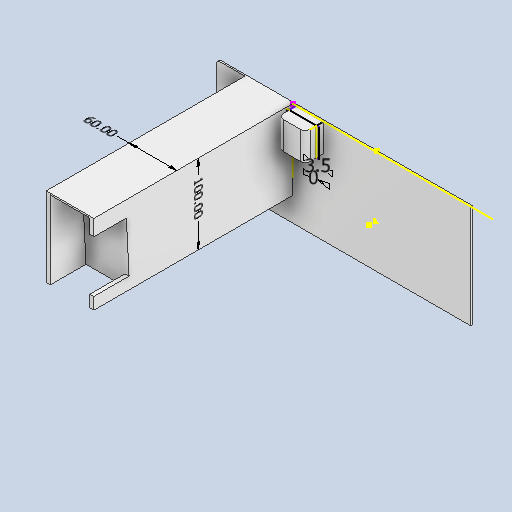
# Autodesk Inventor part: lifting base
Saved by Autodesk Inventor 2025.4 (Build 294407000, 407)
## iProperties
Created: 2026-03-06
Part Number: lifting base
Material: PPS Plastic
Document SubType Name: Modeling
Designer: eslam
Density: 1.637 g/cm^3
Appearance: Smooth - White
Mass: 2489.39 g
Surface Area: 2288.15 cm^2
Volume: 1520.71 cm^3
Author: eslam
Autodesk Inventor part; units mm, degrees
ref_plane "YZ Plane" through (0, 0, 0) normal (1, 0, 0) x (0, 1, 0)
ref_plane "XZ Plane" through (0, 0, 0) normal (0, 1, 0) x (-1, 0, 0)
sketch "Sketch1" plane through (0, 0, 0) normal (0, 0, 1) x (1, 0, 0)
  line L0 (200, 75) -> (-200, 75)
  line L1 (-200, 75) -> (-200, -75)
  line L2 (-200, -75) -> (200, -75)
  line L3 (200, -75) -> (200, 75)
  line L4 (200, 75) -> (-200, -75) construction
  line L5 (-200, 75) -> (200, -75) construction
  point P0 (0, 0)
  dimension "d0" = 400
  dimension "d1" = 150
  constraints: 12 end point, 2 midpoint, 2 parallel, 1 horizontal, 1 perpendicular
  measures "d0" distance of L2.end L1.end
  measures "d1" distance of L1.end L0.end
extrude "Extrusion1" add sketch "Sketch1" along normal blind 2
sketch "Sketch2" plane through (0, 0, 2) normal (0, 0, 1) x (1, 0, 0)
  line L0 (-200, 0) -> (-155, 56.4222) construction
  line L1 (-155, -56.4222) -> (-200, 0) construction
  line L2 (-104.6282, 75) -> (-164.6282, 75)
  line L3 (-164.6282, 75) -> (-164.6282, -25)
  line L4 (-164.6282, -25) -> (-104.6282, -25)
  line L5 (-104.6282, -25) -> (-104.6282, 75)
  line L6 (-104.6282, 75) -> (-164.6282, -25) construction
  line L7 (-164.6282, 75) -> (-104.6282, -25) construction
  line L8 (200, 75) -> (-200, 75) projected
  point P0 (0, 0)
  point P1 (-134.6282, 25)
  dimension "d5" = 60
  dimension "d6" = 100
  dimension "d55" = 0
  constraints: 16 end point, 2 midpoint, 2 parallel, 1 horizontal, 1 perpendicular
  measures "d5" distance of L4.end L3.end
  measures "d6" distance of L3.end L2.end
  measures "d55" distance between parallel lines of L8 L2
extrude "Extrusion2" add sketch "Sketch2" along normal blind 250
sketch "Sketch3" plane through (-104.6282, -25, 2) normal (1, 0, 0) x (0, 0, -1)
  line L0 (0, 0) -> (-250, 0) projected
  line L1 (0, -50) -> (0, 100) projected
  line L2 (0, 100) -> (-250, 100) projected
  line L3 (-250, 0) -> (-250, 100) projected
  line L4 (0, 20) -> (-150, 20)
  line L5 (-150, 80) -> (0, 80)
  line L6 (0, 20) -> (0, 80)
  line L7 (-150, 80) -> (-150, 20)
  point P0 (2, 25)
  dimension "d27" = 20
  dimension "d28" = 20
  constraints: 8 end point, 2 point on line, 1 horizontal, 1 parallel, 1 perpendicular, 1 vertical
  measures "d27" distance between parallel lines of L0 L4
  measures "d28" distance between parallel lines of L5 L2
extrude "Extrusion3" cut sketch "Sketch3" against normal blind 300 contours L4 L7 L5 L1
sketch "Sketch4" plane through (-104.6282, -25, 252) normal (1, 0, 0) x (0, 0, -1)
  line L0 (0, 100) -> (0, 0) projected
  line L1 (0, 80) -> (45, 80)
  line L2 (45, 80) -> (45, 15)
  line L3 (0, 15) -> (0, 80)
  line L4 (45, 15) -> (0, 15)
  line L5 (0, 0) -> (0, 100) projected
  line L6 (0, 15) -> (0, 80)
  point P0 (252, 25)
  dimension "d30" = 65
  dimension "d31" = 15
  dimension "d32" = 45
  dimension "d37" = 65
  constraints: 10 end point, 2 parallel, 2 perpendicular, 2 point on line, 1 collinear, 1 horizontal
  measures "d30" distance of L1.end L2.end
  measures "d31" distance of L0.end L4.end
  measures "d32" distance between parallel lines of L0 L2
  measures "d37" distance of L1.start L3.start
extrude "Extrusion4" cut sketch "Sketch4" against normal blind 55
sketch "Sketch6" plane through (-104.6282, 55, 207) normal (0, -1, 0) x (1, 0, 0)
  line L0 (0, 0) -> (0, 45) projected
  line L1 (0, 0) -> (-55, 0) projected
  line L2 (-55, 0) -> (-55, 45) projected
  line L3 (0, 45) -> (-55, 45) projected
  line L4 (-55, 45) -> (0, 45) projected
  line L5 (0, 45) -> (0, 0)
  line L6 (-5, 45) -> (-5, 0)
  line L7 (-55, 45) -> (-5, 45)
  line L8 (-55, 0) -> (-5, 0)
  line L9 (-55, 45) -> (-55, 0)
  point P0 (104.6282, -207)
  dimension "d40" = 5
  constraints: 10 end point, 3 collinear, 1 parallel, 1 point on line, 1 vertical
  measures "d40" distance between parallel lines of L5 L6
extrude "Extrusion5" cut sketch "Sketch6" against normal blind 18 contours L1 L2 L3 L6
sketch "Sketch7" plane through (-104.6282, -10, 252) normal (0, 1, 0) x (1, 0, 0)
  line L0 (-55, 0) -> (-5, 0) projected
  line L1 (-55, 45) -> (-55, 0) projected
  line L2 (-5, 45) -> (-55, 45) projected
  line L3 (-5, 0) -> (-5, 45) projected
  line L4 (-5, 0) -> (-55, 0)
  line L5 (-55, 0) -> (-55, 45)
  line L6 (-55, 45) -> (-5, 45)
  line L7 (-5, 45) -> (-5, 0)
  point P0 (104.6282, 252)
  constraints: 8 end point, 2 parallel, 1 horizontal, 1 perpendicular
extrude "Extrusion6" cut sketch "Sketch7" against normal through all
sketch "Sketch10" plane through (-159.6282, -25, 252) normal (1, 0, 0) x (0, 0, -1)
  line L0 (45, 98) -> (0, 98) projected
  line L1 (45, 98) -> (45, 0) projected
  line L2 (39.864, 98) -> (45, 0)
  line L3 (45, 0) -> (45, 98)
  line L4 (0, 80) -> (0, 100) projected
  line L5 (45, 98) -> (39.864, 98)
  point P0 (252, 25)
  dimension "d50" = 3
  constraints: 6 end point, 1 parallel, 1 perpendicular, 1 point on line
  measures "d50" angle of L1 L2
extrude "Extrusion7" add sketch "Sketch10" along normal blind 55
fillet "Fillet3" radius 2 3 edges at (-109.6282, 73, 232.068) (-109.6282, -17.5, 207.3931) (-109.6282, 64, 211.6643)
sketch "Sketch11" plane through (0, 0, 2) normal (0, 0, 1) x (1, 0, 0)
  line L0 (-104.6282, -5) -> (-104.6282, 55) projected
  point P0 (0, 0)
  point P1 (-104.6282, 75)
sketch "Sketch12" plane through (-104.6282, -25, 252) normal (1, 0, 0) x (0, 0, -1)
  line L0 (250, 20) -> (100, 20) projected
  line L1 (100, 80) -> (250, 80) projected
  arc A0 (100, 80) -> (100, 20) centre (100, 50) ccw projected
  line L2 (247, 20) -> (250, 20)
  line L3 (247, 80) -> (250, 80)
  line L4 (250, -50) -> (250, 100) projected
  point P0 (252, 25)
  point P1 (250, 22.1792)
  point P2 (250, 77.8208)
  dimension "d57" = 3
  constraints: 4 end point, 4 point on line, 2 collinear
  measures "d57" distance from line of L4 L3.start
extrude "Extrusion8" add sketch "Sketch12" against normal blind 60
ref_plane "Work Plane2" through (-200, 75, 0) normal (0, 1, 0) x (1, 0, 0)
sketch "Sketch15" plane through (-200, 75, 0) normal (0, 1, 0) x (1, 0, 0)
  line L0 (95.3718, -2) -> (95.3718, -252) projected
  line L1 (400, -2) -> (95.3718, -2) projected
  line L2 (100.3718, -11) -> (100.3718, -19)
  line L3 (106.3718, -25) -> (128.3718, -25)
  line L4 (134.3718, -19) -> (134.3718, -11)
  arc A0 (128.3718, -25) -> (134.3718, -19) centre (128.3718, -19) ccw
  arc A1 (100.3718, -19) -> (106.3718, -25) centre (106.3718, -19) ccw
  line L5 (134.3718, -11) -> (100.3718, -11)
  line L6 (100.3718, -11) -> (134.3718, -11)
  line L7 (134.3718, -11) -> (134.3718, -2)
  line L8 (134.3718, -2) -> (100.3718, -2)
  line L9 (100.3718, -2) -> (100.3718, -11)
  point P0 (200, 0)
  point P1 (100.3718, -25)
  point P2 (134.3718, -25)
  dimension "d78" = 14
  dimension "d79" = 34
  dimension "d80" = 6
  dimension "d81" = 5
  constraints: 16 end point, 5 point on line, 4 point on circle, 4 tangent, 3 horizontal, 2 centre point, 2 parallel, 2 perpendicular, 1 equal radius, 1 vertical
  measures "d78" distance of L2.start point (100.372, -25)
  measures "d79" distance of point (100.372, -25) point (134.372, -25)
  measures "d80" radius of A0
  measures "d81" distance between parallel lines of L0 L2
extrude "Extrusion10" add sketch "Sketch15" against normal blind 35 contours L4 A0 L3 A1 L2 L5
sketch "Sketch16" plane through (-200, 40, 0) normal (0, -1, 0) x (1, 0, 0)
  line L0 (128.3718, 25) -> (106.3718, 25) projected
  arc A0 (134.3718, 19) -> (128.3718, 25) centre (128.3718, 19) ccw projected
  arc A1 (106.3718, 25) -> (100.3718, 19) centre (106.3718, 19) ccw projected
  line L1 (134.3718, 11) -> (134.3718, 19) projected
  arc A2 (134.3718, 19) -> (128.3718, 25) centre (128.3718, 19) ccw projected
  line L2 (128.3718, 25) -> (106.3718, 25) projected
  arc A3 (106.3718, 25) -> (100.3718, 19) centre (106.3718, 19) ccw projected
  line L3 (100.3718, 19) -> (100.3718, 11) projected
  line L4 (133.3718, 19) -> (133.3718, 3)
  line L5 (133.3718, 3) -> (101.3718, 3)
  line L6 (101.3718, 3) -> (101.3718, 19)
  arc A4 (106.3718, 24) -> (101.3718, 19) centre (106.3718, 19) ccw
  line L7 (106.3718, 24) -> (128.3718, 24)
  arc A5 (133.3718, 19) -> (128.3718, 24) centre (128.3718, 19) ccw
  line L8 (100.3718, 11) -> (134.3718, 11) projected
  point P0 (200, 0)
  dimension "d85" = 1
  constraints: 8 end point, 4 point on circle, 2 centre point, 3 other
  measures "d85" distance between parallel lines of L1 L4
extrude "Extrusion11" cut sketch "Sketch16" against normal blind 31 contours L8 L6 A4 L7 A5 L4 | L4 L5 L6 L8
fillet "Fillet4" radius 3 1 edges at (-200, -75, 1)
fillet "Fillet5" radius 3 1 edges at (-200, 75, 1)
fillet "Fillet6" radius 3 2 edges at (200, -75, 1) (200, 75, 1)
sketch "Sketch18" plane through (200, -72, 0) normal (1, 0, 0) x (0, 0, -1)
  line L0 (-2, 144) -> (0, 144) projected
  line L1 (-2, 0) -> (-2, 144) projected
  line L2 (0, 0) -> (-2, 0) projected
  line L3 (0, 0) -> (0, 144) projected
  line L4 (-2, 147) -> (-2, 144) projected
  line L5 (-2, 144) -> (0, 144) projected
  line L6 (0, 144) -> (0, 147) projected
  line L7 (0, 147) -> (-2, 147) projected
  line L8 (-2, 0) -> (-2, -3) projected
  line L9 (-2, -3) -> (0, -3) projected
  line L10 (0, -3) -> (0, 0) projected
  line L11 (0, 0) -> (-2, 0) projected
  point P0 (0, 72)
extrude "Extrusion12" cut sketch "Sketch18" against normal blind 50
sketch "Sketch19" plane through (-197, -75, 0) normal (0, -1, 0) x (1, 0, 0)
  line L0 (347, 0) -> (347, 2) projected
  line L1 (0, 2) -> (347, 2) projected
  line L2 (0, 0) -> (0, 2) projected
  line L3 (0, 0) -> (347, 0) projected
  line L4 (0, 2) -> (-3, 2) projected
  line L5 (-3, 2) -> (-3, 0) projected
  line L6 (-3, 0) -> (0, 0) projected
  line L7 (0, 0) -> (0, 2) projected
  point P0 (197, 0)
extrude "Extrusion13" cut sketch "Sketch19" against normal blind 20
fillet "Fillet7" radius 3 2 edges at (150, -55, 1) (150, 75, 1)
fillet "Fillet8" radius 3 1 edges at (-200, -55, 1)
sketch "Sketch20" plane through (-200, 75, 0) normal (0, 1, 0) x (1, 0, 0)
  line L0 (134.3718, -11) -> (134.3718, -19) projected
  line L1 (347, -2) -> (95.3718, -2) projected
  line L2 (134.3718, -11) -> (100, -11)
  line L3 (100, -11) -> (100, -2)
  line L4 (100, -2) -> (134.3718, -2)
  line L5 (134.3718, -2) -> (134.3718, -11)
  point P0 (200, 0)
  constraints: 8 end point, 2 parallel, 1 horizontal, 1 perpendicular, 1 point on line
sketch "Sketch21" plane through (-65.6282, 75, 19) normal (1, 0, 0) x (0, 0, -1)
  line L0 (0, -35) -> (8, -35) projected
  line L1 (17, -100) -> (17, 0) projected
  line L2 (8, -35) -> (17, -35)
  line L3 (17, -35) -> (17, 0)
  line L4 (17, 0) -> (8, 0)
  line L5 (8, 0) -> (8, -35)
  point P0 (19, -75)
  point P1 (17, -22.1792)
  constraints: 8 end point, 2 parallel, 1 horizontal, 1 perpendicular
extrude "Extrusion14" add sketch "Sketch21" against normal blind 37.5
sketch "Sketch22" plane through (-103.1282, 75, 11) normal (0, 0, 1) x (1, 0, 0)
  point P0 (103.1282, -75)
sketch "Sketch23" plane through (-103.1282, 75, 11) normal (0, 0, 1) x (1, 0, 0)
  line L0 (3.5, 0) -> (0, 0) projected
  line L1 (0, 0) -> (3.5, 0)
  line L2 (3.5, 0) -> (3.5, -35)
  line L3 (3.5, -35) -> (0, -35)
  line L4 (0, -35) -> (0, 0)
  line L5 (37.5, 0) -> (41, 0)
  line L6 (41, 0) -> (41, -35)
  line L7 (41, -35) -> (37.5, -35)
  line L8 (37.5, -35) -> (37.5, 0)
  line L9 (37.5, 0) -> (37.5, -35) projected
  point P0 (103.1282, -75)
  dimension "d100" = 3.5
  dimension "d101" = 0
  constraints: 16 end point, 4 parallel, 2 horizontal, 2 perpendicular
  measures "d100" distance of L6.end L7.end
  measures "d101" distance between parallel lines of L9 L8
sketch "Sketch24" plane through (-200, 40, 0) normal (0, -1, 0) x (1, 0, 0)
  line L0 (133.3718, 11) -> (101.3718, 11) projected
  line L1 (117.3718, 11) -> (117.3718, 2) construction
  line L2 (134.3718, 2) -> (96.8718, 2) projected
  line L3 (134.3718, 19) -> (134.3718, 2) projected
  line L4 (134.3718, 11) -> (134.3718, 2)
  line L5 (100.3718, 11) -> (100.3718, 2)
  line L6 (96.8718, 11) -> (100.3718, 11)
  line L7 (100.3718, 11) -> (100.3718, 2)
  line L8 (100.3718, 2) -> (96.8718, 2)
  line L9 (96.8718, 2) -> (96.8718, 11)
  point P0 (200, 0)
  point P1 (96.8718, 2)
  constraints: 14 end point, 2 parallel, 2 symmetric about line, 2 vertical, 1 horizontal, 1 midpoint, 1 perpendicular, 1 point on line
extrude "Extrusion17" cut sketch "Sketch24" against normal through all
sketch "Sketch26" plane through (-200, 40, 0) normal (0, -1, 0) x (1, 0, 0)
  line L0 (101.3718, 11) -> (101.3718, 19) projected
  line L1 (101.3718, 17) -> (103.3718, 17)
  line L2 (133.3718, 11) -> (101.3718, 11) projected
  circle A0 centre (103.3718, 17) radius 2
  line L3 (133.3718, 17) -> (131.6357, 17)
  circle A1 centre (103.3718, 17) radius 1.25
  line L4 (103.3718, 18.25) -> (101.3718, 18.25)
  line L5 (101.3718, 18.25) -> (101.3718, 15.75)
  line L6 (101.3718, 15.75) -> (103.3718, 15.75)
  line L7 (103.3718, 15.75) -> (103.3718, 18.25)
  circle A2 centre (130.6718, 17) radius 2
  circle A3 centre (130.6718, 17) radius 1.25
  line L8 (133.3718, 19) -> (133.3718, 11) projected
  line L9 (130.6718, 18.25) -> (133.3718, 18.25)
  line L10 (133.3718, 18.25) -> (133.3718, 15.25)
  line L11 (133.3718, 15.25) -> (130.6718, 15.25)
  line L12 (130.6718, 15.25) -> (130.6718, 18.25)
  point P0 (200, 0)
  point P1 (132.233, 18.25)
  point P2 (131.64, 15.25)
  point P3 (101.8105, 15.75)
  point P4 (101.8105, 18.25)
  dimension "d116" = 2.5
  dimension "d118" = 2.5
  dimension "d119" = 27.3
  dimension "d112" = 6
  dimension "d113" = 4
  dimension "d117" = 4
  constraints: 20 end point, 4 horizontal, 4 parallel, 3 coincident, 3 point on line, 2 centre point, 2 perpendicular, 2 vertical alignment, 1 horizontal alignment, 1 midpoint, 4 other
  measures "d112" distance between parallel lines of L2 L1
  measures "d113" diameter of A0
  measures "d117" diameter of A2
extrude "Extrusion18" add sketch "Sketch26" against normal blind 10
extrude "Extrusion19" cut sketch "Sketch26" against normal blind 10 contours A1 L7 L1 | L1 L7 A1 | L7 A1 | A3 L12 | L12 A3
thread "Thread3" size "M2.5x0.45" class "6H" standard "ANSI Metric M Profile" length 72
thread "Thread4" size "M2.5x0.45" class "6H" standard "ANSI Metric M Profile" length 72
sketch "Sketch28" plane through (150, -72, 0) normal (1, 0, 0) x (0, 0, -1)
  line L0 (0, 144) -> (0, 20) projected
  line L1 (-2, 20) -> (0, 20)
  line L2 (0, 20) -> (0, 144)
  line L3 (0, 144) -> (-2, 144)
  line L4 (-2, 144) -> (-2, 20)
  point P0 (0, 72)
  constraints: 8 end point, 2 parallel, 1 horizontal, 1 perpendicular
extrude "Extrusion21" add sketch "Sketch28" along normal blind 50
sketch "Sketch29" plane through (0, 0, 2) normal (0, 0, 1) x (1, 0, 0)
  line L0 (200, 72) -> (200, -52) projected
  line L1 (200, 72) -> (200, -52)
  line L2 (200, 10) -> (160.5, 10)
  line L3 (160.5, 10) -> (160.5, 16)
  line L4 (160.5, 16) -> (115.5, 16)
  line L5 (115.5, 16) -> (115.5, 4)
  line L6 (115.5, 4) -> (160.5, 4)
  line L7 (160.5, 4) -> (160.5, 16)
  point P0 (0, 0)
  dimension "d136" = 39.5
  dimension "d137" = 6
  dimension "d138" = 45
  dimension "d139" = 12
  constraints: 14 end point, 2 horizontal, 2 parallel, 2 vertical, 1 midpoint, 1 perpendicular
  measures "d136" distance of L2.start L2.end
  measures "d137" distance of L2.end L3.end
  measures "d138" distance of L6.end L5.end
  measures "d139" distance of L5.end L4.end
sketch "Sketch31" plane through (0, 0, 2) normal (0, 0, 1) x (1, 0, 0)
  line L0 (147, 75) -> (-65.6282, 75) projected
  line L1 (119.1362, 75) -> (234.7266, 75)
  line L2 (234.7266, 75) -> (234.7266, -58.1498)
  line L3 (234.7266, -58.1498) -> (119.1362, -58.1498)
  line L4 (119.1362, -58.1498) -> (119.1362, 75)
  point P0 (0, 0)
  constraints: 8 end point, 2 parallel, 1 horizontal, 1 perpendicular, 1 point on line
extrude "Extrusion24" cut sketch "Sketch31" against normal blind 10
body "Solid1"
